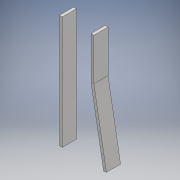
# Autodesk Inventor part: 導軌
Saved by Autodesk Inventor 2017 (Build 210142000, 142)
## iProperties
Part Number: 導軌
Material: 一般
Document SubType Name: Modeling
Designer: Blin
Density: 1 g/cm^3
Appearance: 預設
Author: Blin
Autodesk Inventor part; units mm, degrees
ref_plane "YZ Plane" through (0, 0, 0) normal (1, 0, 0) x (0, 1, 0)
ref_plane "XZ Plane" through (0, 0, 0) normal (0, 1, 0) x (-1, 0, 0)
ref_plane "XY Plane" through (0, 0, 0) normal (0, 0, 1) x (1, 0, 0)
sketch "草圖1" plane through (0, 0, 0) normal (0, 1, 0) x (-1, 0, 0)
  line L0 (0, 0) -> (10, 0)
  line L1 (10, 0) -> (10, -400)
  line L2 (10, -400) -> (0, -400)
  line L3 (0, -400) -> (0, 0)
  line L4 (-112, 0) -> (-102, 0)
  line L5 (-102, 0) -> (-102, -150)
  line L6 (-102, -150) -> (-112, -150)
  line L7 (-112, -150) -> (-112, 0)
  line L8 (-102, -150) -> (-111.846, -148.2517)
  line L9 (-111.846, -148.2517) -> (-156.2359, -398.2517)
  line L10 (-156.2359, -398.2517) -> (-146.3899, -400)
  line L11 (-146.3899, -400) -> (-102, -150)
  dimension "d0" = 102
  dimension "d1" = 10
  dimension "d2" = 10
  dimension "d3" = 10
  dimension "d4" = 150
  dimension "d5" = 400
  dimension "d6" = 250
  constraints: 24 end point, 6 parallel, 3 perpendicular, 2 horizontal, 1 point on line
  measures "d0" distance between parallel lines of L3 L5
  measures "d1" distance of L1.end L2.end
  measures "d2" distance of L4.start L4.end
  measures "d3" distance of L9.end L10.end
  measures "d4" distance of L4.end L5.end
  measures "d5" distance of L0.end L1.end
  measures "d6" distance from line of L6 L10.end
extrude "擠出1" add sketch "草圖1" along normal blind 50
fillet "圓角1" radius 10 1 edges at (102, 25, -150)
